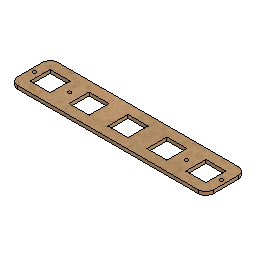
Leds nivel accidente capa1 (Autodesk Fusion 360 design; units mm, degrees)
Autodesk Fusion 360 part; units mm, degrees
sketch "Sketch1" plane through (0, 0, 0) normal (0, 0, 1) x (1, 0, 0)
  line L0 (-9, 9) -> (9, 9)
  line L1 (9, 9) -> (9, -9)
  line L2 (9, -9) -> (-9, -9)
  line L3 (-9, -9) -> (-9, 9)
  line L4 (-9, 9) -> (9, -9) construction
  line L5 (9, 9) -> (-9, -9) construction
  line L6 (-81, 18) -> (81, 18)
  line L7 (88, 11) -> (88, -11)
  line L8 (81, -18) -> (-81, -18)
  line L9 (-88, -11) -> (-88, 11)
  line L10 (-88, 18) -> (88, -18) construction
  line L11 (88, 18) -> (-88, -18) construction
  arc A0 (-81, 18) -> (-88, 11) centre (-81, 11) ccw
  arc A1 (-88, -11) -> (-81, -18) centre (-81, -11) ccw
  arc A2 (81, -18) -> (88, -11) centre (81, -11) ccw
  arc A3 (88, 11) -> (81, 18) centre (81, 11) ccw
  line L12 (0, 0) -> (0, 18) construction
  circle A4 centre (-84, 0) radius 1.5
  line L13 (-79, 9) -> (-61, 9)
  line L14 (-79, -9) -> (-79, 9)
  line L15 (-61, -9) -> (-79, -9)
  line L16 (-61, 9) -> (-61, -9)
  line L17 (-44, 9) -> (-26, 9)
  line L18 (-44, -9) -> (-44, 9)
  line L19 (-26, -9) -> (-44, -9)
  line L20 (-26, 9) -> (-26, -9)
  line L21 (26, 9) -> (44, 9)
  line L22 (26, -9) -> (26, 9)
  line L23 (44, -9) -> (26, -9)
  line L24 (44, 9) -> (44, -9)
  line L25 (61, 9) -> (79, 9)
  line L26 (61, -9) -> (61, 9)
  line L27 (79, -9) -> (61, -9)
  line L28 (79, 9) -> (79, -9)
  circle A5 centre (84, 0) radius 1.5
  circle A6 centre (-52.5, 0) radius 1.5
  circle A7 centre (52.5, 0) radius 1.5
  dimension "d22" = 18
  dimension "d23" = 18
  dimension "d28" = 176
  dimension "d29" = 36
  dimension "d30" = 7
  dimension "d35" = 3
  dimension "d36" = 4
  dimension "d37" = 18
  dimension "d44" = 35
  dimension "d45" = 0
  dimension "d60" = 3
  dimension "d61" = 8.5
  constraint perpendicular L0 L1
  constraint parallel L0 L2
  constraint parallel L1 L3
  constraint horizontal L0
  constraint coincident L4 L12.start
  constraint coincident L5 L12.start
  constraint coincident L12.start origin
  constraint perpendicular L6 L7
  constraint parallel L6 L8
  constraint parallel L7 L9
  constraint horizontal L6
  constraint coincident L10 L12.start
  constraint coincident L11 L12.start
  constraint coincident L10.start L6
  constraint coincident L10.start L9
  constraint tangent L6 A0
  constraint tangent L9 A0
  constraint coincident L11.end L9
  constraint coincident L11.end L8
  constraint tangent L9 A1
  constraint tangent L8 A1
  constraint equal A0 A1
  constraint coincident L10.end L8
  constraint coincident L10.end L7
  constraint tangent L8 A2
  constraint tangent L7 A2
  constraint equal A0 A2
  constraint coincident L11.start L7
  constraint coincident L11.start L6
  constraint tangent L7 A3
  constraint tangent L6 A3
  constraint equal A0 A3
  constraint midpoint L6 L12.end
  constraint symmetric L12 A4 A5
  constraint symmetric L12 A6 A7
  measures "d22" distance of L1.end L2.end
  measures "d23" distance of L0.end L1.end
  measures "d28" distance of L10.end L11.end
  measures "d29" distance of L11.start L10.end
  measures "d30" radius of A0
  measures "d35" diameter of A4
  measures "d36" distance of L9 A4.centre
  measures "d37" distance of L6 A4.centre
  measures "d60" diameter of A6
  measures "d61" distance of L16 A6.centre
extrude "Extrude6" add sketch "Sketch1" along normal blind 3
equation "d44 = 17 mm + 18 mm"
equation "d61 = ( 17 / 2 ) * 1 mm"
